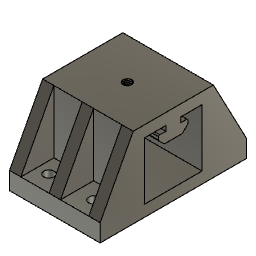
Stage+Mount (Autodesk Fusion 360 design; units mm, degrees)
Autodesk Fusion 360 part; units mm, degrees
note: some values were not read from the file. Set by a fixed rule: the direction of a hole.
sketch "Stage" plane through (0, 0, 0) normal (0, 0, 1) x (1, 0, 0) in component "Stage Mount"
  line L0 (-7.9, -50) -> (-7.9, 50)
  line L1 (7.9, 50) -> (7.9, -50)
  line L2 (-11.9, 50) -> (-11.9, -50)
  line L3 (11.9, -50) -> (11.9, 50)
  line L4 (20, -75) -> (-20, -75)
  line L5 (-20, -75) -> (-20, 75)
  line L6 (-20, 75) -> (20, 75)
  line L7 (20, 75) -> (20, -75)
  line L8 (-11.9, 50) -> (-7.9, 50)
  line L9 (7.9, 50) -> (11.9, 50)
  line L10 (7.9, -50) -> (11.9, -50)
  line L11 (-11.9, -50) -> (-7.9, -50)
  dimension "d1" = 15.8
  dimension "d3" = 23.8
  dimension "d4" = 40
  dimension "d5" = 150
  constraint horizontal L4
  constraint perpendicular L4 L5
  constraint perpendicular L0 L8
  constraint perpendicular L3 L9
  constraint perpendicular L3 L10
  constraint perpendicular L0 L11
  measures "d1" distance of L0.end L1.start
  measures "d3" distance of L2.end L3.start
  measures "d4" distance of L5.end L6.end
  measures "d5" distance of L4.end L5.end
sketch "Sketch2" plane through (0, 0, 0) normal (1, 0, 0) x (0, 1, 0) in component "Stage Mount"
  line L0 (0, 5) -> (12.7, 5)
  line L1 (0, 5) -> (-12.7, 5)
  line L2 (-12.7, 5) -> (-12.7, 30.4)
  line L3 (12.7, 5) -> (12.7, 30.4)
  line L4 (12.7, 30.4) -> (-12.7, 30.4)
  line L5 (0, 35.4) -> (17.7, 35.4)
  line L6 (0, 35.4) -> (-17.7, 35.4)
  line L7 (-17.7, 35.4) -> (-50, 5)
  line L8 (-50, 5) -> (-50, 0)
  line L9 (-50, 0) -> (50, 0)
  line L10 (50, 0) -> (50, 5)
  line L11 (50, 5) -> (17.7, 35.4)
  line L12 (50, 5) -> (12.7, 5)
  line L13 (-12.7, 5) -> (-50, 5)
  line L14 (17.7, 35.4) -> (17.7, 5)
  line L15 (-17.7, 35.4) -> (-17.7, 5)
  dimension "d8" = 25.4
  dimension "d11" = 17.7
  dimension "d12" = 17.7
  constraint perpendicular L1 L2
  constraint perpendicular L0 L3
  constraint perpendicular L3 L5
  constraint perpendicular L6 L8
  constraint perpendicular L8 L9
  constraint perpendicular L9 L10
  constraint perpendicular L3 L12
  constraint perpendicular L8 L13
  constraint coincident L12 L14.end
  constraint perpendicular L12 L14
  constraint coincident L13 L15.end
  constraint perpendicular L13 L15
  measures "d8" distance of L1.end L2.end
  measures "d11" distance of L5.start L5.end
  measures "d12" distance of L5.start L6.end
extrude "Extrude1" add sketch "Sketch2" along normal mid plane 40 contours L0 L1 L8 L9 L10 L12 L13 | L2 L3 L4 L5 L6 L12 L13 L14 L15 makes body 1 in component "Stage Mount"
extrude "Extrude2" add sketch "Sketch2" along normal mid plane 5 contours L11 L12 L14 | L7 L13 L15 bodies 1 in component "Stage Mount"
extrude "Extrude3" add sketch "Sketch2" along normal blind 5 from surface at 15 contours L11 L12 L14 | L7 L13 L15 bodies 1 in component "Stage Mount"
extrude "Extrude4" add sketch "Sketch2" against normal blind 5 from surface at -15 contours L11 L12 L14 | L7 L13 L15 bodies 1 in component "Stage Mount"
sketch "Sketch3" plane through (0, 0, 0) normal (0, 0, 1) x (1, 0, 0) in component "Stage Mount"
  line L0 (9.9, -25) -> (-9.9, -25)
  line L1 (-9.9, 25) -> (9.9, 25)
  line L2 (9.9, 42.5) -> (-9.9, 42.5)
  line L3 (-9.9, -42.5) -> (9.9, -42.5)
hole "Hole1" at (9.9, 42.5, 0) at (-9.9, 42.5, 0) at (-9.9, 25, 0) at (9.9, 25, 0) at (-9.9, -25, 0) at (9.9, -25, 0) at (-9.9, -42.5, 0) at (9.9, -42.5, 0) direction (0, 0, 1) diameter 4 end up to surface (5 mm away) bodies 1 in component "Stage Mount"
chamfer "Chamfer1" distance 1 angle 45 8 edges at (-20, -12.7, 17.7) (-20, 0, 30.4) (-20, 12.7, 17.7) (-20, 0, 5) (20, 0, 30.4) (20, -12.7, 17.7) (20, 0, 5) (20, 12.7, 17.7) on bodies 1 in component "Stage Mount"
copy_body "CopyPasteBodies1" bodies 1 makes body 2 in component "Stage Mount"
extrude "Extrude5" add 1 faces at (-3.0107, -7.7327, 0) along direction (0, 0, -1) blind 1 separate body on bodies 2 makes body 3 in component "Stage Mount"
sketch "Sketch4" plane through (0, 0, -1) normal (0, 0, -1) x (1, 0, 0) in component "Stage Mount"
  circle A0 centre (-9.9, 42.5) radius 2
  circle A1 centre (-9.9, 25) radius 2
  circle A2 centre (-9.9, -25) radius 2
  circle A3 centre (9.9, -42.5) radius 2
  circle A4 centre (-9.9, -42.5) radius 2
  circle A5 centre (9.9, -25) radius 2
  circle A6 centre (9.9, 25) radius 2
  circle A7 centre (9.9, 42.5) radius 2
  line L0 (-20, -50) -> (20, -50)
  line L1 (20, -50) -> (20, 50)
  line L2 (20, 50) -> (-20, 50)
  line L3 (-20, 50) -> (-20, -50)
  circle A8 centre (9.9, 42.5) radius 2
  circle A9 centre (-9.9, 42.5) radius 2
  circle A10 centre (-9.9, 25) radius 2
  circle A11 centre (9.9, 25) radius 2
  circle A12 centre (9.9, -25) radius 2
  circle A13 centre (9.9, -42.5) radius 2
  circle A14 centre (-9.9, -42.5) radius 2
  circle A15 centre (-9.9, -25) radius 2
  line L4 (9.9, -42.5) -> (9.9, -44.5)
  line L5 (9.9, -42.5) -> (9.9, 27)
  line L6 (9.9, 27) -> (-20, 27)
  line L7 (9.9, 23) -> (-20, 23)
  line L8 (9.9, -27) -> (-20, -27)
  line L9 (9.9, -23) -> (-20, -23)
  line L10 (9.9, -40.5) -> (-20, -40.5)
  line L11 (9.9, -44.5) -> (-20, -44.5)
  line L12 (9.9, 27) -> (9.9, 44.5)
  line L13 (9.9, 44.5) -> (-20, 44.5)
  line L14 (9.9, 40.5) -> (-20, 40.5)
  constraint concentric A7 A8
  constraint concentric A0 A9
  constraint concentric A1 A10
  constraint concentric A6 A11
  constraint concentric A5 A12
  constraint concentric A3 A13
  constraint concentric A4 A14
  constraint concentric A2 A15
  constraint coincident A3.centre A13.centre
  constraint coincident A13 L4.end
  constraint vertical L4
  constraint coincident A6 L5.end
  constraint parallel L4 L5
  constraint coincident L3 L6.end
  constraint perpendicular L3 L6
  constraint coincident A11 L7.start
  constraint coincident L5 L7.start
  constraint coincident L3 L7.end
  constraint tangent A11 L7
  constraint coincident L5 L8.start
  constraint coincident A12 L8.start
  constraint coincident L3 L8.end
  constraint tangent A12 L8
  constraint coincident L5 L9.start
  constraint coincident A12 L9.start
  constraint coincident L3 L9.end
  constraint tangent A12 L9
  constraint coincident L5 L10.start
  constraint coincident A13 L10.start
  constraint coincident L3 L10.end
  constraint tangent A3 L10
  constraint perpendicular L3 L10
  constraint coincident L3 L11.end
  constraint tangent A3 L11
  constraint perpendicular L3 L11
  constraint coincident A8 L12.end
  constraint perpendicular L6 L12
  constraint coincident L3 L13.end
  constraint tangent A8 L13
  constraint coincident A8 L14.start
  constraint coincident L12 L14.start
  constraint coincident L3 L14.end
  constraint tangent A8 L14
extrude "Extrude6" cut sketch "Sketch4" against normal blind 1 contours A0 A7 A8 A9 L13 L14 | A0 L3 A9 L13 L14 | A1 A6 A10 A11 L6 L7 | A1 L3 A10 L6 L7 | A2 A5 A12 A15 L8 L9 | A2 L3 A15 L8 L9 | A4 L3 A14 L10 L11 | A3 A4 A13 A14 L10 L11 bodies 3 in component "Stage Mount"
sketch "Sketch5" plane through (0, 0, 0) normal (1, 0, 0) x (0, 1, 0) in component "Stage Mount"
  line L0 (0, 5) -> (12.7, 5)
  line L1 (0, 5) -> (-12.7, 5)
  line L2 (-12.7, 5) -> (-12.7, 30.4)
  line L3 (12.7, 5) -> (12.7, 30.4)
  line L4 (12.7, 30.4) -> (-12.7, 30.4)
  line L5 (0, 0) -> (-24.7995, 0)
  line L6 (0, 0) -> (25, 0)
  line L7 (25, 0) -> (32.2995, 0)
  line L8 (-24.7995, 0) -> (-32.2995, 0)
  line L9 (-32.2995, 0) -> (-32.2995, 7.75)
  line L10 (32.2995, 0) -> (32.2995, 7.75)
  line L11 (0, 35.4) -> (-17.7, 35.4)
  line L12 (-17.7, 35.4) -> (-32.2995, 7.75)
  line L13 (-17.7, 35.4) -> (-17.7, 7.75)
  line L14 (0, 35.4) -> (17.7, 35.4)
  line L15 (17.7, 35.4) -> (17.7, 7.75)
  line L16 (17.7, 7.75) -> (32.2995, 7.75)
  line L17 (32.2995, 7.75) -> (17.7, 35.4)
  line L18 (-17.7, 7.75) -> (-32.2995, 7.75)
  line L19 (6.5, 28.2) -> (6.5, 26.2)
  line L20 (-6.5, 28.2) -> (-6.5, 26.2)
  line L21 (0, 23.7) -> (-4, 23.7)
  line L22 (0, 23.7) -> (4, 23.7)
  line L23 (4, 23.7) -> (6.5, 26.2)
  line L24 (-4, 23.7) -> (-6.5, 26.2)
  line L25 (0, 28.2) -> (3.25, 28.2)
  line L26 (3.25, 28.2) -> (3.25, 30.4)
  line L27 (-3.25, 28.2) -> (-3.25, 30.4)
  line L28 (0, 28.2) -> (-3.25, 28.2)
  line L29 (-3.25, 28.2) -> (-6.5, 28.2)
  line L30 (3.25, 28.2) -> (6.5, 28.2)
  dimension "d40" = 7.5
  constraint coincident L5.start L6.start
  constraint parallel L5 L8
  constraint perpendicular L8 L9
  constraint perpendicular L7 L10
  constraint perpendicular L10 L16
  constraint perpendicular L9 L18
  constraint coincident L4 L26.end
  constraint coincident L4 L27.end
  measures "d40" distance of L5.end L8.end
extrude "Extrude7" add sketch "Sketch5" along normal mid plane 40 separate body contours L4 L25 L26 L27 L28 | L19 L20 L21 L22 L23 L24 L25 L28 L29 L30 | L5 L6 L7 L8 L9 L10 L11 L13 L14 L15 L16 L18 makes body 4 in component "Stage Mount"
hole "Hole2" at (9.9, -25, 0) at (-9.9, -25, 0) at (-9.9, 25, 0) at (9.9, 25, 0) direction (0, 0, 1) diameter 4.5 depth 10 tip angle 180 bodies 4 in component "Stage Mount"
extrude "Extrude8" add sketch "Sketch5" along normal blind 5 from surface at 15 contours L12 L13 L18 | L15 L16 L17 bodies 4 in component "Stage Mount"
extrude "Extrude9" add sketch "Sketch5" along normal mid plane 5 contours L12 L13 L18 | L15 L16 L17 bodies 4 in component "Stage Mount"
extrude "Extrude10" add sketch "Sketch5" against normal blind 5 from surface at -15 contours L12 L13 L18 | L15 L16 L17 bodies 4 in component "Stage Mount"
sketch "Sketch6" plane through (0, 0, 0) normal (1, 0, 0) x (0, 1, 0) in component "Stage Mount"
  line L0 (12.7, -12.7) -> (-12.7, -12.7)
  line L1 (-12.7, -12.7) -> (-12.7, 12.7)
  line L2 (-12.7, 12.7) -> (12.7, 12.7)
  line L3 (12.7, 12.7) -> (12.7, -12.7)
  line L4 (-3.25, 10.5) -> (-3.25, 12.7)
  line L5 (3.25, 10.5) -> (3.25, 12.7)
  line L6 (-3.25, 10.5) -> (-6.5, 10.5)
  line L7 (3.25, 10.5) -> (6.5, 10.5)
  line L8 (6.5, 10.5) -> (6.5, 8.5)
  line L9 (-6.5, 10.5) -> (-6.5, 8.5)
  line L10 (0, 6) -> (-4, 6)
  line L11 (0, 6) -> (4, 6)
  line L12 (4, 6) -> (6.5, 8.5)
  line L13 (-4, 6) -> (-6.5, 8.5)
  line L14 (-10.5, 3.25) -> (-12.7, 3.25)
  line L15 (-10.5, 3.25) -> (-10.5, 6.5)
  line L16 (-6, 4) -> (-8.5, 6.5)
  line L17 (-10.5, 6.5) -> (-8.5, 6.5)
  line L18 (-6, 0) -> (-6, 4)
  line L19 (-6, 0) -> (-6, -4)
  line L20 (-6, -4) -> (-8.5, -6.5)
  line L21 (-10.5, -6.5) -> (-8.5, -6.5)
  line L22 (-10.5, -3.25) -> (-12.7, -3.25)
  line L23 (-10.5, -3.25) -> (-10.5, -6.5)
  line L24 (-3.25, -10.5) -> (-3.25, -12.7)
  line L25 (-3.25, -10.5) -> (-6.5, -10.5)
  line L26 (-4, -6) -> (-6.5, -8.5)
  line L27 (-6.5, -10.5) -> (-6.5, -8.5)
  line L28 (0, -6) -> (-4, -6)
  line L29 (0, -6) -> (4, -6)
  line L30 (4, -6) -> (6.5, -8.5)
  line L31 (6.5, -10.5) -> (6.5, -8.5)
  line L32 (3.25, -10.5) -> (3.25, -12.7)
  line L33 (3.25, -10.5) -> (6.5, -10.5)
  line L34 (10.5, -3.25) -> (12.7, -3.25)
  line L35 (10.5, -3.25) -> (10.5, -6.5)
  line L36 (6, -4) -> (8.5, -6.5)
  line L37 (10.5, -6.5) -> (8.5, -6.5)
  line L38 (6, 0) -> (6, -4)
  line L39 (6, 0) -> (6, 4)
  line L40 (6, 4) -> (8.5, 6.5)
  line L41 (10.5, 6.5) -> (8.5, 6.5)
  line L42 (10.5, 3.25) -> (12.7, 3.25)
  line L43 (10.5, 3.25) -> (10.5, 6.5)
  line L44 (15.2, 15.2) -> (-15.2, 15.2)
  line L45 (-15.2, 15.2) -> (-15.2, -15.2)
  line L46 (-15.2, -15.2) -> (15.2, -15.2)
  line L47 (15.2, -15.2) -> (15.2, 15.2)
  dimension "d81" = 30.4
  dimension "d82" = 30.4
  dimension "d94" = 2.2
  dimension "d95" = 2
  dimension "d96" = 3.25
  dimension "d97" = 3.5355
  dimension "d98" = 4
  dimension "d99" = 25.4
  dimension "d100" = 6.7
  dimension "d101" = 6.5
  constraint coincident L2 L4.end
  constraint coincident L2 L5.end
  constraint horizontal L44
  constraint perpendicular L44 L45
  constraint parallel L44 L46
  constraint parallel L45 L47
  measures "d81" distance of L45.end L46.end
  measures "d82" distance of L44.end L45.end
  measures "d94" distance of L4.start L4.end
  measures "d95" distance of L6.end L9.end
  measures "d96" distance of L4.start L6.end
  measures "d97" distance of L9.end L10.end
  measures "d98" distance of L10.start L10.end
  measures "d99" distance of L1.end L2.end
  measures "d100" distance of L2 L10
  measures "d101" distance of L4 L5
extrude "Extrude11" add sketch "Sketch6" along normal blind 2.5 separate body contours L0 L24 L25 L26 L27 L28 L29 L30 L31 L32 L33 | L3 L34 L35 L36 L37 L38 L39 L40 L41 L42 L43 | L1 L14 L15 L16 L17 L18 L19 L20 L21 L22 L23 | L2 L4 L5 L6 L7 L8 L9 L10 L11 L12 L13 | L44 L45 L46 L47 makes body 5 in component "Stage Mount"
fillet "Fillet1" radius 2.5 4 edges at (1.25, -15.2, 15.2) (1.25, -15.2, -15.2) (1.25, 15.2, -15.2) (1.25, 15.2, 15.2) on bodies 5 in component "Stage Mount"
hole "Hole3" at (0, 0, 35.4) direction (0, 0, -1) diameter 3.416 depth 18 tip angle 180 bodies 4 in component "Stage Mount"
thread "Thread1" "ANSI Unified Screw Threads 0.164(#8) 8-32 UNC 2B" major diameter 4.1656 minor diameter 3.4163 pitch 0.7937 angle 60 modelled right hand crest width 0.2341 on face at (0.1701, -1.6995, 31.5) crest through (1.7082, 0, 35.2016) on bodies 4 in component "Stage Mount"
fillet "Fillet2" radius 0.5 6 edges at (0, -6.5, 28.2) (0, -6.5, 26.2) (0, -4, 23.7) (0, 4, 23.7) (0, 6.5, 28.2) (0, 6.5, 26.2) on bodies 4 in component "Stage Mount"
move_body "Move1" bodies 5 to x (1, 0, 0) y (0, 1, 0) z (0, 0, 1) at (68, 0, 0) in component "Stage Mount"
copy_body "CopyPasteBodies2" bodies 5 makes body 6 in component "Stage Mount"
move_body "Move2" bodies 6 to x (1, 0, 0) y (0, 1, 0) z (0, 0, 1) at (10, 0, 0) in component "Stage Mount"
fillet "Fillet3" radius 0.5 24 edges at (79.25, -6.5, 10.5) (79.25, -6.5, 8.5) (79.25, -4, 6) (79.25, 4, 6) (79.25, 6.5, 8.5) (79.25, 6.5, 10.5) (79.25, 8.5, 6.5) (79.25, 10.5, 6.5) (79.25, 6, 4) (79.25, 6, -4) (79.25, 8.5, -6.5) (79.25, 10.5, -6.5) (79.25, -10.5, 6.5) (79.25, -8.5, 6.5) (79.25, -6, 4) (79.25, -6, -4) (79.25, -8.5, -6.5) (79.25, -10.5, -6.5) (79.25, -6.5, -10.5) (79.25, -6.5, -8.5) (79.25, -4, -6) (79.25, 4, -6) (79.25, 6.5, -8.5) (79.25, 6.5, -10.5) on bodies 6 in component "Stage Mount"
component "Stage Mount" placed x (1, 0, 0) y (0, 1, 0) z (0, 0, 1) at (0, 0, 0)
hidden bodies 1 2 3 5 6
named bodies: "Stage Mount", "T-Slot Test", "T-Slot Test Fillet"
